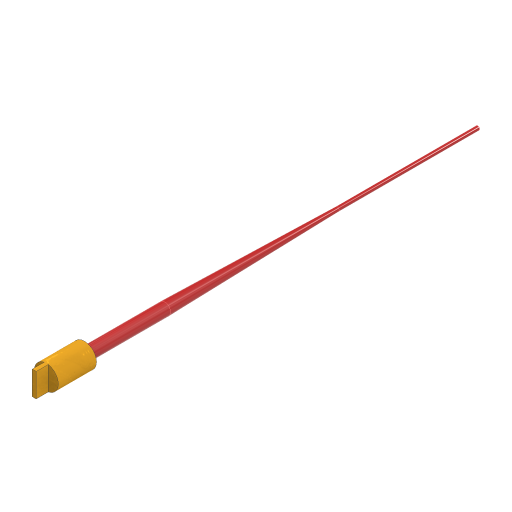
# Autodesk Inventor part: Лазер маленький 2
Saved by Autodesk Inventor 2023 (Build 270158000, 158)
## iProperties
Created: 2022-11-06
Part Number: Лазер маленький 2
Material: Типовые
Document SubType Name: Modeling
Designer: Admin
Density: 1 g/cm^3
Appearance: По умолчанию
Author: Admin
Autodesk Inventor part; units mm, degrees
ref_plane "YZ Plane" through (0, 0, 0) normal (1, 0, 0) x (0, 1, 0)
ref_plane "XY Plane" through (0, 0, 0) normal (0, 0, 1) x (1, 0, 0)
sketch "Эскиз1" plane through (0, 0, 0) normal (0, 0, 1) x (1, 0, 0)
  circle A0 centre (0, 0) radius 3
  dimension "d0" = 6
  constraints: 1 centre point, 1 coincident
  measures "d0" diameter of A0
extrude "Выдавливание1" add sketch "Эскиз1" along normal blind 9.5
sketch "Эскиз2" plane through (0, 0, 9.5) normal (0, 0, 1) x (1, 0, 0)
  circle A0 centre (0, 0) radius 3 projected
  line L0 (-0.5, 2.958) -> (-0.5, -2.958)
  line L1 (0.5, -2.958) -> (0.5, 2.958)
  line L2 (0, 0) -> (0, 0.4981) construction
  dimension "d3" = 1
  constraints: 6 end point, 4 point on circle, 2 vertical, 1 parallel, 1 other
  measures "d3" distance between parallel lines of L0 L1
extrude "Выдавливание2" add sketch "Эскиз2" along normal blind 3 contours L1 A0 L0
sketch "Эскиз3" plane through (0, 0, 0) normal (0, 0, -1) x (-1, 0, 0)
  circle A0 centre (0, 0) radius 2
  dimension "d6" = 4
  constraints: 1 centre point, 1 coincident
  measures "d6" diameter of A0
extrude "Выдавливание3" cut sketch "Эскиз3" against normal blind 2
sketch "Эскиз5" plane through (0, 0, 2) normal (0, 0, -1) x (-1, 0, 0)
  circle A0 centre (0, 0) radius 1.5
  dimension "d11" = 3
  constraints: 1 centre point, 1 coincident
  measures "d11" diameter of A0
extrude "Выдавливание5" add sketch "Эскиз5" along normal blind 22 separate body
sketch "Эскиз6" plane through (0, 0, -20) normal (0, 0, -1) x (-1, 0, 0)
  circle A0 centre (0, 0) radius 1.5 projected
ref_plane "РабПлоскость1" through (0, 0, -20) normal (0, 1, 0) x (-1, 0, 0)
sketch "Эскиз7" plane through (0, 0, -20) normal (0, 1, 0) x (-1, 0, 0)
  line L0 (0, 0) -> (0, -43)
  line L1 (1.5, 22) -> (1.5, 0) projected
  point P0 (0, 20)
  dimension "d14" = 43
  constraints: 2 end point, 1 coincident, 1 vertical
  measures "d14" distance of L0.start L0.end
ref_plane "РабПлоскость2" through (0, 0, -63) normal (0, 0, -1) x (-1, 0, 0)
sketch "Эскиз8" plane through (0, 0, -63) normal (0, 0, -1) x (-1, 0, 0)
  circle A0 centre (0, 0) radius 0.5
  point P0 (0, 0)
  dimension "d15" = 1
  constraints: 1 centre point, 1 coincident
  measures "d15" diameter of A0
loft "Лофт1" add profiles "Эскиз8" bodies 2 section 1 edges at (1.5, 0, -20)
extrude "Выдавливание6" add sketch "Эскиз8" along normal blind 35 bodies 2
